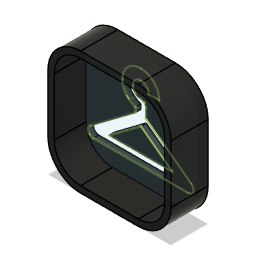
Trellis Keycap Hanger (Autodesk Fusion 360 design; units mm, degrees)
Autodesk Fusion 360 part; units mm, degrees
sketch "Sketch1" plane through (0, 0, 0) normal (0, 0, 1) x (1, 0, 0)
  line L0 (2.72, 5) -> (-2.72, 5)
  line L1 (-5, 2.72) -> (-5, -2.72)
  line L2 (-2.72, -5) -> (2.72, -5)
  line L3 (5, -2.72) -> (5, 2.72)
  line L4 (5, 5) -> (-5, -5) construction
  line L5 (-5, 5) -> (5, -5) construction
  arc A0 (5, 2.72) -> (2.72, 5) centre (2.72, 2.72) ccw
  arc A1 (2.72, -5) -> (5, -2.72) centre (2.72, -2.72) ccw
  arc A2 (-5, -2.72) -> (-2.72, -5) centre (-2.72, -2.72) ccw
  arc A3 (-2.72, 5) -> (-5, 2.72) centre (-2.72, 2.72) ccw
  line L6 (-2.72, -5.2) -> (2.72, -5.2)
  arc A4 (2.72, -5.2) -> (5.2, -2.72) centre (2.72, -2.72) ccw
  line L7 (5.2, -2.72) -> (5.2, 2.72)
  arc A5 (5.2, 2.72) -> (2.72, 5.2) centre (2.72, 2.72) ccw
  line L8 (2.72, 5.2) -> (-2.72, 5.2)
  arc A6 (-2.72, 5.2) -> (-5.2, 2.72) centre (-2.72, 2.72) ccw
  line L9 (-5.2, 2.72) -> (-5.2, -2.72)
  arc A7 (-5.2, -2.72) -> (-2.72, -5.2) centre (-2.72, -2.72) ccw
  line L10 (-2.72, -5.8) -> (2.72, -5.8)
  arc A8 (2.72, -5.8) -> (5.8, -2.72) centre (2.72, -2.72) ccw
  line L11 (5.8, -2.72) -> (5.8, 2.72)
  arc A9 (5.8, 2.72) -> (2.72, 5.8) centre (2.72, 2.72) ccw
  line L12 (2.72, 5.8) -> (-2.72, 5.8)
  arc A10 (-2.72, 5.8) -> (-5.8, 2.72) centre (-2.72, 2.72) ccw
  line L13 (-5.8, 2.72) -> (-5.8, -2.72)
  arc A11 (-5.8, -2.72) -> (-2.72, -5.8) centre (-2.72, -2.72) ccw
  dimension "d1" = 10
  dimension "d2" = 10
  dimension "d3" = 2.28
  dimension "d4" = 0.2
  dimension "d5" = 0.8
  constraint horizontal L0
  constraint perpendicular L0 L1
  constraint parallel L0 L2
  constraint parallel L1 L3
  constraint coincident L4 origin
  constraint coincident L5 origin
  constraint coincident L4.start L0
  constraint coincident L4.start L3
  constraint tangent L0 A0
  constraint tangent L3 A0
  constraint coincident L5.end L3
  constraint coincident L5.end L2
  constraint tangent L3 A1
  constraint tangent L2 A1
  constraint equal A0 A1
  constraint coincident L4.end L2
  constraint coincident L4.end L1
  constraint tangent L2 A2
  constraint tangent L1 A2
  constraint equal A0 A2
  constraint coincident L5.start L1
  constraint coincident L5.start L0
  constraint tangent L1 A3
  constraint tangent L0 A3
  constraint equal A0 A3
  measures "d1" distance of L4.end L5.end
  measures "d2" distance of L5.start L4.end
  measures "d3" radius of A0
extrude "Extrude1" add sketch "Sketch1" along normal blind 3 contours L10 A8 L11 A9 L12 A10 L13 A11 makes body 1
extrude "Extrude2" add sketch "Sketch1" against normal blind 0.5 contours L0 L1 L2 L3 A0 A1 A2 A3 | L6 A4 L7 A5 L8 A6 L9 A7 | L10 A8 L11 A9 L12 A10 L13 A11 bodies 1
sketch "Sketch3" plane through (0, 0, 0) normal (0, 0, 1) x (1, 0, 0)
  line L0 (-2.72, -5.2) -> (2.72, -5.2)
  arc A0 (2.72, -5.2) -> (5.2, -2.72) centre (2.72, -2.72) ccw
  line L1 (5.2, -2.72) -> (5.2, 2.72)
  arc A1 (5.2, 2.72) -> (2.72, 5.2) centre (2.72, 2.72) ccw
  line L2 (2.72, 5.2) -> (-2.72, 5.2)
  arc A2 (-2.72, 5.2) -> (-5.2, 2.72) centre (-2.72, 2.72) ccw
  line L3 (-5.2, 2.72) -> (-5.2, -2.72)
  arc A3 (-5.2, -2.72) -> (-2.72, -5.2) centre (-2.72, -2.72) ccw
  arc A4 (1.6946, 2.4851) -> (-0.0405, 4.2202) centre (-0.0405, 2.4851) ccw
  line L4 (1.6946, 2.4851) -> (0.7031, 2.4851)
  arc A5 (0.7031, 2.4851) -> (-0.0405, 3.2287) centre (-0.0405, 2.4851) ccw
  arc A6 (-0.0405, 3.2287) -> (-0.7841, 2.4851) centre (-0.0405, 2.4851) ccw
  arc A7 (-0.7841, 2.4851) -> (-0.0405, 1.7416) centre (-0.0405, 2.4851) ccw
  spline S0 degree 3 poles (-0.0405, 1.7416) (0.2322, 1.7416) (0.4553, 1.5185) (0.4553, 1.2458) knots 0 0 0 0 1 1 1 1
  line L5 (0.4553, 1.2458) -> (0.4553, 0.3783)
  line L6 (0.4553, 0.3783) -> (4.7186, -2.8192)
  arc A8 (4.4211, -3.7115) -> (4.7186, -2.8192) centre (4.4211, -3.2158) ccw
  line L7 (4.4211, -3.7115) -> (-4.502, -3.7115)
  arc A9 (-4.7995, -2.8192) -> (-4.502, -3.7115) centre (-4.502, -3.2158) ccw
  line L8 (-4.7995, -2.8192) -> (-0.5362, 0.3783)
  line L9 (-0.5362, 0.3783) -> (-0.5362, 0.8244)
  arc A10 (-1.7755, 2.4851) -> (-0.5362, 0.8244) centre (-0.0405, 2.4872) ccw
  arc A11 (-0.0405, 4.2202) -> (-1.7755, 2.4851) centre (-0.0405, 2.4851) ccw
  line L10 (-0.0405, -0.4892) -> (-3.0148, -2.72)
  line L11 (-3.0148, -2.72) -> (2.9339, -2.72)
  line L12 (2.9339, -2.72) -> (-0.0405, -0.4892)
extrude "Extrude5" cut sketch "Sketch3" against normal blind 0.5 contours A4 L4 A5 A6 A7 S0 L5 L6 A8 L7 A9 L8 L9 A10 A11 bodies 1 makes body 2 at (-4.0336, 0.4839, -0.5)
extrude "Extrude6" add sketch "Sketch3" against normal blind 0.5 separate body contours A4 L4 A5 A6 A7 S0 L5 L6 A8 L7 A9 L8 L9 A10 A11 makes body 3
sketch "Sketch2" plane through (0, 0, 0) normal (0, 0, 1) x (1, 0, 0)
  line L0 (-2.72, -5.2) -> (2.72, -5.2)
  arc A0 (2.72, -5.2) -> (5.2, -2.72) centre (2.72, -2.72) ccw
  line L1 (5.2, -2.72) -> (5.2, 2.72)
  arc A1 (5.2, 2.72) -> (2.72, 5.2) centre (2.72, 2.72) ccw
  line L2 (2.72, 5.2) -> (-2.72, 5.2)
  arc A2 (-2.72, 5.2) -> (-5.2, 2.72) centre (-2.72, 2.72) ccw
  line L3 (-5.2, 2.72) -> (-5.2, -2.72)
  arc A3 (-5.2, -2.72) -> (-2.72, -5.2) centre (-2.72, -2.72) ccw
  arc A4 (-1.656, 2.2908) -> (0.0167, 3.9635) centre (0.0167, 2.2908) cw
  line L4 (-1.656, 2.2908) -> (-0.7001, 2.2908)
  arc A5 (-0.7001, 2.2908) -> (0.0167, 3.0076) centre (0.0167, 2.2908) cw
  arc A6 (0.0167, 3.0076) -> (0.7336, 2.2908) centre (0.0167, 2.2908) cw
  arc A7 (0.7336, 2.2908) -> (0.0167, 1.5739) centre (0.0167, 2.2908) cw
  spline S0 degree 3 poles (0.0167, 1.5739) (-0.2461, 1.5739) (-0.4612, 1.3588) (-0.4612, 1.096) knots 0 0 0 0 1 1 1 1
  line L5 (-0.4612, 1.096) -> (-0.4612, 0.2596)
  line L6 (-0.4612, 0.2596) -> (-4.5713, -2.823)
  arc A8 (-4.2845, -3.6832) -> (-4.5713, -2.823) centre (-4.2845, -3.2053) cw
  line L7 (-4.2845, -3.6832) -> (4.318, -3.6832)
  arc A9 (4.6048, -2.823) -> (4.318, -3.6832) centre (4.318, -3.2053) cw
  line L8 (4.6048, -2.823) -> (0.4947, 0.2596)
  line L9 (0.4947, 0.2596) -> (0.4947, 0.6897)
  arc A10 (1.6895, 2.2908) -> (0.4947, 0.6897) centre (0.0167, 2.2927) cw
  arc A11 (0.0167, 3.9635) -> (1.6895, 2.2908) centre (0.0167, 2.2908) cw
  line L10 (0.0167, -0.5768) -> (2.8842, -2.7274)
  line L11 (2.8842, -2.7274) -> (-2.8508, -2.7274)
  line L12 (-2.8508, -2.7274) -> (0.0167, -0.5768)
extrude "Extrude3" [suppressed]
extrude "Extrude4" [suppressed]
named bodies: "Keycap", "Keycap (1)"
